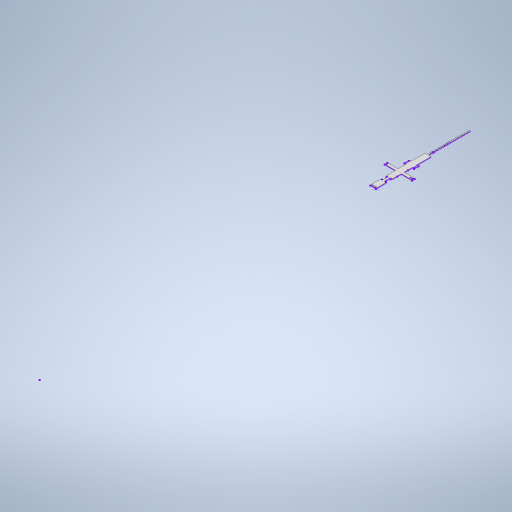
# Autodesk Inventor part: Middle Finger Part
Saved by Autodesk Inventor 2023.1 (Build 271208000, 208)
## iProperties
Created: 2022-09-21
Part Number: Middle Finger Part
Material: Generic
Document SubType Name: Modeling
Designer: lxpe222
Density: 1 g/cm^3
Appearance: Default
Author: lxpe222
Autodesk Inventor part; units mm, degrees
ref_plane "YZ Plane" through (0, 0, 0) normal (1, 0, 0) x (0, 1, 0)
ref_plane "XZ Plane" through (0, 0, 0) normal (0, 1, 0) x (-1, 0, 0)
ref_plane "XY Plane" through (0, 0, 0) normal (0, 0, 1) x (1, 0, 0)
sketch "Sketch1" plane through (0, 0, 0) normal (0, 1, 0) x (-1, 0, 0)
  line L0 (-9.2572, 22.5392) -> (-9.2572, 5.2228)
  line L1 (-9.2588, 35.8907) -> (-9.2588, 54.0006)
  line L2 (-7.7588, 55.5006) -> (0.6256, 55.5006)
  line L3 (2.1256, 54.0006) -> (2.1256, 36.0144)
  circle A0 centre (-0.0494, 53.5306) radius 1.175
  circle A1 centre (-6.816, 53.5306) radius 1.175
  line L4 (-9.2572, 22.5392) -> (-7.5421, 22.5392)
  line L5 (-5.2699, 24.8114) -> (-5.2699, 33.6185)
  line L6 (-7.5421, 35.8907) -> (-9.2588, 35.8907)
  line L7 (2.1256, 36.0144) -> (0.4105, 36.0144)
  line L8 (-1.8617, 33.7422) -> (-1.8617, 24.9778)
  line L9 (0.4105, 22.7056) -> (2.1256, 22.7056)
  arc A2 (0.4105, 36.0144) -> (-1.8617, 33.7422) centre (0.4105, 33.7422) ccw
  arc A3 (-1.8617, 24.9778) -> (0.4105, 22.7056) centre (0.4105, 24.9778) ccw
  arc A4 (-7.5421, 22.5392) -> (-5.2699, 24.8114) centre (-7.5421, 24.8114) ccw
  arc A5 (-5.2699, 33.6185) -> (-7.5421, 35.8907) centre (-7.5421, 33.6185) ccw
  line L10 (2.1256, 5.2228) -> (22.3981, 5.2228)
  line L11 (23.8981, 3.7228) -> (23.8981, 1.4538)
  line L12 (22.3981, -0.0462) -> (2.3981, -0.0462)
  line L13 (-9.2572, 5.2228) -> (-29.2572, 5.2228)
  line L14 (-30.7572, 3.7228) -> (-30.7572, 1.4538)
  line L15 (-29.2572, -0.0462) -> (-9.2572, -0.0462)
  line L16 (2.3981, -16.3797) -> (5.0881, -16.3797)
  line L17 (6.0881, -17.3797) -> (6.0881, -24.3797)
  line L18 (5.0881, -25.3797) -> (2.3981, -25.3797)
  line L19 (-9.2572, -16.3797) -> (-11.9472, -16.3797)
  line L20 (-12.9472, -17.3797) -> (-12.9472, -24.3797)
  line L21 (-11.9472, -25.3797) -> (-9.2572, -25.3797)
  circle A6 centre (-3.2163, 53.4806) radius 0.85
  circle A7 centre (-25.4, 2.6538) radius 1.2
  circle A8 centre (-29.025, 2.6538) radius 0.825
  circle A9 centre (21.7231, 2.6538) radius 1.2
  line L22 (-9.2572, -0.0462) -> (-9.2572, -16.3797)
  line L23 (2.1256, 5.2228) -> (2.1256, 22.7056)
  line L24 (2.3981, -16.3797) -> (2.3981, -0.0462)
  arc A10 (2.1256, 54.0006) -> (0.6256, 55.5006) centre (0.6256, 54.0006) ccw
  arc A11 (-7.7588, 55.5006) -> (-9.2588, 54.0006) centre (-7.7588, 54.0006) ccw
  arc A12 (22.3981, -0.0462) -> (23.8981, 1.4538) centre (22.3981, 1.4538) ccw
  arc A13 (23.8981, 3.7228) -> (22.3981, 5.2228) centre (22.3981, 3.7228) ccw
  arc A14 (-30.7572, 1.4538) -> (-29.2572, -0.0462) centre (-29.2572, 1.4538) ccw
  arc A15 (-29.2572, 5.2228) -> (-30.7572, 3.7228) centre (-29.2572, 3.7228) ccw
  line L25 (-3.1006, -58.0771) -> (-4.1675, -56.1771)
  line L26 (-3.1006, -58.0771) -> (-0.5618, -58.1074) construction
  line L27 (-4.1983, -59.9271) -> (-3.1006, -58.0771)
  line L28 (-3.1573, -63.8271) -> (-4.1983, -61.9271)
  line L29 (-4.2026, -65.6771) -> (-3.1573, -63.8271)
  line L30 (-3.1444, -69.5771) -> (-4.2026, -67.6771)
  line L31 (-4.2286, -71.4271) -> (-3.1444, -69.5771)
  line L32 (-3.1748, -75.3271) -> (-4.2286, -73.4271)
  line L33 (-4.2398, -77.1771) -> (-3.1748, -75.3271)
  line L34 (-3.189, -81.0771) -> (-4.2398, -79.1771)
  line L35 (-4.2405, -82.9271) -> (-3.189, -81.0771)
  line L36 (-3.1609, -86.8265) -> (-4.2405, -84.9271)
  line L37 (-4.3046, -88.6765) -> (-3.1609, -86.8265)
  line L38 (-3.1955, -92.5764) -> (-4.3046, -90.6765)
  line L39 (-4.3306, -94.4264) -> (-3.1955, -92.5764)
  line L40 (-3.2465, -98.4318) -> (-4.3306, -96.4264)
  line L41 (-2.7028, -60.5238) -> (-1.6676, -62.3738)
  line L42 (-1.7097, -58.6238) -> (-2.7028, -60.5238)
  line L43 (-2.6949, -66.2738) -> (-1.6645, -68.1238)
  line L44 (-1.6676, -64.3738) -> (-2.6949, -66.2738)
  line L45 (-2.7162, -72.0238) -> (-1.6901, -73.8738)
  line L46 (-1.6645, -70.1238) -> (-2.7162, -72.0238)
  line L47 (-2.7304, -77.7738) -> (-1.7072, -79.6238)
  line L48 (-1.6901, -75.8738) -> (-2.7304, -77.7738)
  line L49 (-2.732, -83.5238) -> (-1.688, -85.3738)
  line L50 (-1.7072, -81.6238) -> (-2.732, -83.5238)
  line L51 (-2.7571, -89.2738) -> (-1.6815, -91.1238)
  line L52 (-1.688, -87.3738) -> (-2.7571, -89.2738)
  line L53 (-2.5461, -95.1105) -> (-1.4416, -96.9605)
  line L54 (-1.5878, -93.2105) -> (-2.5461, -95.1105)
  line L55 (-1.5878, -93.2105) -> (-1.6815, -93.1238)
  line L56 (-4.3046, -88.6765) -> (-4.3046, -90.6765)
  line L57 (-4.3306, -94.4264) -> (-4.3306, -96.4264)
  line L58 (-4.2398, -77.1771) -> (-4.2398, -79.1771)
  line L59 (-4.2405, -82.9271) -> (-4.2405, -84.9271)
  line L60 (-4.1675, -53.7002) -> (-4.1675, -56.1771)
  line L61 (-4.1983, -59.9271) -> (-4.1983, -61.9271)
  line L62 (-4.2026, -65.6771) -> (-4.2026, -67.6771)
  line L63 (-4.2286, -71.4271) -> (-4.2286, -73.4271)
  line L64 (-1.6676, -64.3738) -> (-1.6676, -62.3738)
  line L65 (-1.6645, -70.1238) -> (-1.6645, -68.1238)
  line L66 (-1.6901, -75.8738) -> (-1.6901, -73.8738)
  line L67 (-1.7072, -81.6238) -> (-1.7072, -79.6238)
  line L68 (-1.6815, -93.1238) -> (-1.6815, -91.1238)
  line L69 (-1.688, -87.3738) -> (-1.688, -85.3738)
  line L70 (-3.372, -120.8894) -> (-4.3473, -122.6628)
  line L71 (-3.372, -120.8894) -> (-4.425, -119.0541)
  line L72 (-3.2465, -98.4318) -> (-4.3098, -99.808)
  line L73 (-3.2659, -115.1473) -> (-4.425, -117.0541)
  line L74 (-3.2659, -115.1473) -> (-4.2167, -113.3098)
  line L75 (-3.1633, -109.4364) -> (-4.2167, -111.3067)
  line L76 (-3.1633, -109.4364) -> (-4.2167, -107.5567)
  line L77 (-3.2112, -103.6888) -> (-4.2167, -105.5567)
  line L78 (-3.2112, -103.6888) -> (-4.313, -101.808)
  line L79 (-2.4945, -100.8807) -> (-1.4416, -98.9605)
  line L80 (-2.4945, -100.8807) -> (-1.4416, -102.7105)
  line L81 (-2.4926, -106.6875) -> (-1.4822, -108.4602)
  line L82 (-2.4926, -106.6875) -> (-1.4416, -104.7105)
  line L83 (-2.5888, -112.3127) -> (-1.5892, -114.2097)
  line L84 (-2.5888, -112.3127) -> (-1.4822, -110.4613)
  line L85 (-2.7673, -117.9845) -> (-1.712, -120.2397)
  line L86 (-2.7673, -117.9845) -> (-1.5892, -116.2097)
  line L87 (-4.3098, -99.808) -> (-4.313, -101.808)
  line L88 (-1.4416, -96.9605) -> (-1.4416, -98.9605)
  line L89 (-1.4416, -102.7105) -> (-1.4416, -104.7105)
  line L90 (-1.4822, -108.4602) -> (-1.4822, -110.4613)
  line L91 (-4.2167, -107.5567) -> (-4.2167, -105.5567)
  line L92 (-4.2167, -111.3067) -> (-4.2167, -113.3098)
  line L93 (-1.5892, -114.2097) -> (-1.5892, -116.2097)
  line L94 (-4.425, -117.0541) -> (-4.425, -119.0541)
  line L95 (2.3981, -53.2502) -> (2.3981, -25.3797)
  line L96 (-9.2572, -25.3797) -> (-9.2572, -53.7002)
  line L97 (-9.2572, -53.7002) -> (-4.1675, -53.7002)
  circle A16 centre (-11.292, -23.3797) radius 0.5
  circle A17 centre (-11.292, -18.3797) radius 0.5
  circle A18 centre (-11.292, -20.8797) radius 0.5
  circle A19 centre (4.4328, -18.3797) radius 0.5
  circle A20 centre (4.4328, -20.8797) radius 0.5
  circle A21 centre (4.4328, -23.3797) radius 0.5
  line L98 (-4.3473, -122.6628) -> (-4.425, -122.8041)
  line L99 (-3.4136, -132.3891) -> (-4.3889, -134.1626)
  line L100 (-3.4136, -132.3891) -> (-4.4666, -130.5538)
  line L101 (-3.396, -126.7927) -> (-4.425, -124.8041)
  line L102 (-3.396, -126.7927) -> (-4.4666, -128.5538)
  line L103 (-2.8724, -129.5355) -> (-1.8315, -131.3699)
  line L104 (-2.8724, -129.5355) -> (-1.8191, -127.6199)
  line L105 (-2.8278, -123.7381) -> (-1.712, -121.8714)
  line L106 (-2.8278, -123.7381) -> (-1.8191, -125.6199)
  line L107 (-4.425, -122.8041) -> (-4.425, -124.8041)
  line L108 (-1.8191, -125.6199) -> (-1.8191, -127.6199)
  line L109 (-4.4666, -128.5538) -> (-4.4666, -130.5538)
  line L110 (-1.712, -121.8714) -> (-1.712, -120.2397)
  line L111 (-1.8315, -131.3699) -> (-1.8315, -133.1348)
  line L112 (-1.8315, -133.1348) -> (-1.8315, -136.784)
  line L113 (-4.3889, -134.1626) -> (-4.3889, -136.784)
  line L114 (-1.8315, -136.784) -> (-4.3889, -136.784)
  line L115 (-1.7097, -58.6238) -> (-1.7097, -53.2502)
  line L116 (-1.7097, -53.2502) -> (2.3981, -53.2502)
  arc A22 (5.0881, -25.3797) -> (6.0881, -24.3797) centre (5.0881, -24.3797) ccw
  arc A23 (6.0881, -17.3797) -> (5.0881, -16.3797) centre (5.0881, -17.3797) ccw
  arc A24 (-11.9472, -16.3797) -> (-12.9472, -17.3797) centre (-11.9472, -17.3797) ccw
  arc A25 (-12.9472, -24.3797) -> (-11.9472, -25.3797) centre (-11.9472, -24.3797) ccw
  point P0 (-9.2588, 55.5006)
  point P1 (2.1256, 55.5006)
  point P2 (-6.9279, 18.3671)
  point P3 (-6.9323, 25.0551)
  point P4 (23.8981, -0.0462)
  point P5 (23.8981, 5.2228)
  point P6 (-30.7572, -0.0462)
  point P7 (-30.7572, 5.2228)
  point P8 (6.0881, -25.3797)
  point P9 (6.0881, -16.3797)
  point P10 (-12.9472, -25.3797)
  point P11 (-12.9472, -16.3797)
  point P12 (-4.1675, 717.4283)
  point P13 (-3.6778, -62.8771)
  point P14 (-3.7007, -85.8768)
  point P15 (-3.75, -91.6265)
  point P16 (-1.9939, -96.0355)
  point P17 (-3.68, -64.7521)
  point P18 (-9.2572, 13.881)
  point P19 (-9.2572, -8.2129)
  point P20 (-10.6022, -25.3797)
  point P21 (3.7431, -25.3797)
  point P22 (3.7431, -16.3797)
  dimension "d276" = 2.4
  dimension "d277" = 2.4
  dimension "d280" = 1.5
  dimension "d281" = 2.35
  dimension "d282" = 2.35
  dimension "d284" = 1.65
  dimension "d286" = 1.7
  dimension "d288" = 0.795
  dimension "d289" = 0.795
  dimension "d290" = 1.17
  dimension "d291" = 1.6
  dimension "d292" = 1.575
  dimension "d293" = 1.5
  dimension "d294" = 1.5
  dimension "d296" = 0.975
  dimension "d297" = 2.175
  dimension "d304" = 120
  dimension "d305" = 120
  dimension "d316" = 2
  dimension "d317" = 2
  dimension "d318" = 2
  dimension "d319" = 2
  dimension "d320" = 2
  dimension "d321" = 2
  dimension "d322" = 2
  dimension "d323" = 2
  dimension "d324" = 2
  dimension "d325" = 2
  dimension "d326" = 2
  dimension "d327" = 2
  dimension "d329" = 2
  dimension "d330" = 2
  dimension "d331" = 2
  dimension "d332" = 2.0032
  dimension "d333" = 2
  dimension "d334" = 2
  dimension "d338" = 3.75
  dimension "d339" = 3.75
  dimension "d340" = 3.75
  dimension "d341" = 3.75
  dimension "d342" = 3.75
  dimension "d343" = 3.75
  dimension "d344" = 3.75
  dimension "d345" = 3.75
  dimension "d346" = 3.75
  dimension "d347" = 3.75
  dimension "d348" = 3.75
  dimension "d349" = 3.75
  dimension "d350" = 3.75
  dimension "d351" = 3.75
  dimension "d352" = 1.85
  dimension "d353" = 1.85
  dimension "d354" = 1.85
  dimension "d355" = 1.85
  dimension "d356" = 1.85
  dimension "d357" = 1.85
  dimension "d358" = 1.85
  dimension "d359" = 1.85
  dimension "d360" = 1.85
  dimension "d361" = 1.85
  dimension "d362" = 1.85
  dimension "d363" = 1.85
  dimension "d364" = 1.85
  dimension "d365" = 1.85
  constraints: 235 end point, 63 parallel, 28 point on circle, 28 tangent, 27 point on line, 26 centre point, 13 vertical, 10 midpoint, 9 equal radius, 9 perpendicular, 6 horizontal, 1 collinear
  measures "d276" diameter of A7
  measures "d277" diameter of A9
  measures "d280" radius of A10
  measures "d281" diameter of A0
  measures "d282" diameter of A1
  measures "d284" diameter of A8
  measures "d286" diameter of A6
  measures "d288" distance edge to line of A1 L2
  measures "d289" distance edge to line of A0 L2
  measures "d290" distance edge to line of A6 L2
  measures "d293" radius of A12
  measures "d294" radius of A14
  measures "d296" distance edge to line of A9 L11
  measures "d297" distance from line of L3 A0.centre
  measures "d304" angle of L26 L25
  measures "d305" angle of L27 L26
  measures "d316" distance of L44.start L41.end
  measures "d317" distance of L27.start L28.end
  measures "d318" distance of L29.start L30.end
  measures "d319" distance of L46.start L43.end
  measures "d320" distance of L31.start L32.end
  measures "d321" distance of L48.start L45.end
  measures "d322" distance of L33.start L34.end
  measures "d323" distance of L50.start L47.end
  measures "d324" distance of L35.start L36.end
  measures "d325" distance of L52.start L49.end
  measures "d326" distance of L37.start L38.end
  measures "d327" distance of L55.end L51.end
  measures "d329" distance of L39.start L40.end
  measures "d330" distance from line of point (-3.678, -62.877) L41
  measures "d331" distance between parallel lines of L30 L43
  measures "d332" distance between parallel lines of L32 L45
  measures "d333" distance between parallel lines of L34 L47
  measures "d334" distance from line of point (-3.701, -85.877) L49
  measures "d338" vertical distance of L53.end L54.start
  measures "d339" distance of L38.end L39.start
  measures "d340" distance of L51.end L52.start
  measures "d341" vertical distance of L50.start L49.end
  measures "d342" distance of L37.start L36.end
  measures "d343" distance of L34.end L35.start
  measures "d344" vertical distance of L48.start L47.end
  measures "d345" distance of L32.end L33.start
  measures "d346" vertical distance of L30.end L31.start
  measures "d347" vertical distance of L46.start L45.end
  measures "d348" distance of L44.start L43.end
  measures "d349" distance of L28.end L29.start
  measures "d350" vertical distance of L42.start L41.end
  measures "d351" vertical distance of L25.end L27.start
  measures "d352" vertical distance of L27.start L25.start
  measures "d353" vertical distance of L29.start L28.start
  measures "d354" vertical distance of L41.start L41.end
  measures "d355" vertical distance of L44.end L43.end
  measures "d356" vertical distance of L31.start L30.start
  measures "d357" vertical distance of L45.end L46.end
  measures "d358" vertical distance of L33.start L32.start
  measures "d359" vertical distance of L48.end L47.end
  measures "d360" vertical distance of L34.start L35.start
  measures "d361" vertical distance of L50.end L49.end
  measures "d362" vertical distance of L52.end L51.end
  measures "d363" vertical distance of L36.start L37.start
  measures "d364" vertical distance of L39.start L38.start
  measures "d365" vertical distance of L54.end L53.end
extrude "Extrusion8" add sketch "Sketch1" along normal blind 1
body "Solid3"
